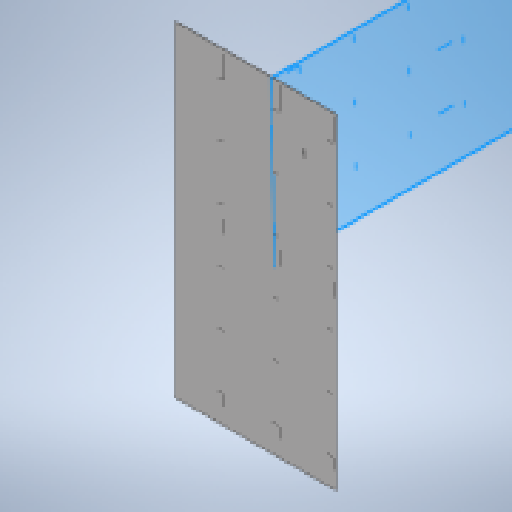
# Autodesk Inventor part: GBK 1211 shield 2
Saved by Autodesk Inventor 2026.2 (Build 302298000, 298)
## iProperties
Created: 2026-04-17
Part Number: GBK 1211 shield 2
Material: Steel
Document SubType Name: Sheet Metal
Designer: pokla
Density: 7.85 g/cm^3
Sheet Metal Rule: Default_mm
Appearance: Default
Mass: 138487 g
Surface Area: 88564.8 cm^2
Volume: 17641.6 cm^3
Sheet Metal Width: 0,000 mm
Sheet Metal Length: 0,000 mm
Sheet Metal Area: 0,000 mm^2
Stock Number: 1211
Author: admin
Autodesk Inventor part; units mm, degrees
ref_plane "YZ Plane" through (0, 0, 0) normal (1, 0, 0) x (0, 1, 0)
ref_plane "XZ Plane" through (0, 0, 0) normal (0, 1, 0) x (-1, 0, 0)
ref_plane "XY Plane" through (0, 0, 0) normal (0, 0, 1) x (1, 0, 0)
sketch "Sketch1" plane through (0, 0, 0) normal (0, 0, 1) x (1, 0, 0)
  line L0 (740, -1490) -> (-740, -1490)
  line L1 (-740, -1490) -> (-740, 1490)
  line L2 (-740, 1490) -> (740, 1490)
  line L3 (740, 1490) -> (740, -1490)
  line L4 (740, -1490) -> (-740, 1490) construction
  line L5 (-740, -1490) -> (740, 1490) construction
  point P0 (0, 0)
  dimension "d0" = 1480
  dimension "d1" = 2980
  measures "d0" distance of L1.end L2.end
  measures "d1" distance of L0.end L1.end
extrude "Plate1" add sketch "Sketch1" along normal blind 4
sketch "Sketch2" plane through (0, 0, 4) normal (0, 0, 1) x (1, 0, 0)
  line L0 (698.6722, 1247.3333) -> (651.6843, 1247.3333) projected
  line L1 (198.8008, 1247.3333) -> (151.8129, 1247.3333) projected
  line L2 (-301.0706, 1247.3333) -> (-348.0585, 1247.3333) projected
  line L3 (-301.0706, 750.6667) -> (-348.0585, 750.6667) projected
  line L4 (198.8008, 750.6667) -> (151.8129, 750.6667) projected
  line L5 (698.6722, 750.6667) -> (651.6843, 750.6667) projected
  line L6 (698.6722, 254) -> (651.6843, 254) projected
  line L7 (698.6722, -242.6667) -> (651.6843, -242.6667) projected
  line L8 (698.6722, -739.3333) -> (651.6843, -739.3333) projected
  line L9 (698.6722, -1236) -> (651.6843, -1236) projected
  line L10 (-301.0706, -242.6667) -> (-348.0585, -242.6667) projected
  line L11 (-301.0706, -739.3333) -> (-348.0585, -739.3333) projected
  line L12 (-301.0706, -1236) -> (-348.0585, -1236) projected
  line L13 (198.8008, -1236) -> (151.8129, -1236) projected
  line L14 (198.8008, -739.3333) -> (151.8129, -739.3333) projected
  line L15 (198.8008, -242.6667) -> (151.8129, -242.6667) projected
  line L16 (198.8008, 254) -> (151.8129, 254) projected
  line L17 (-290.0035, -1243.5) -> (-290.0035, -1340.5) projected
  line L18 (210.1251, -1243.5) -> (210.1251, -1340.5) projected
  line L19 (710.2537, -1243.5) -> (710.2537, -1340.5) projected
  line L20 (710.2537, 1454.5) -> (710.2537, 1250.8333) projected
  line L21 (210.1251, 1454.5) -> (210.1251, 1250.8333) projected
  line L22 (-290.0035, 1454.5) -> (-290.0035, 1250.8333) projected
  line L23 (-301.0706, 254) -> (-348.0585, 254) projected
  line L24 (710.2537, 149.5) -> (710.2537, 24.5) projected
  line L25 (210.1251, 149.5) -> (210.1251, 24.5) projected
  line L26 (-290.0035, 149.5) -> (-290.0035, 24.5) projected
  line L27 (453.1111, 1069.606) -> (453.1111, 711.9156) construction
  line L28 (453.1111, 711.9156) -> (421.8469, 711.9156) construction
  line L29 (421.8469, 711.9156) -> (421.8469, 1069.606) construction
  line L30 (421.8469, 1069.606) -> (453.1111, 1069.606) construction
  point P0 (0, 0)
  constraints: 2 other
mark "Mark1"
equation "\"d0\" = Лист_ширина"
equation "\"d2\" = Thickness"
equation "\"BendRadius\" = Thickness"
equation "\"BendReliefWidth\" = Thickness"
equation "\"BendReliefDepth\" = 0.5 * Thickness"
equation "\"CornerReliefSize\" = 4 * Thickness"
equation "\"MinimumRemnant\" = 2 * Thickness"
equation "\"TransitionRadius\" = BendRadius"
equation "\"JacobiRadiusSize\" = BendRadius"
equation "\"GapSize\" = Thickness"
equation "\"Лист_ширина\" = 1480"
equation "\"Thickness\" = 4"
body "Solid1"
